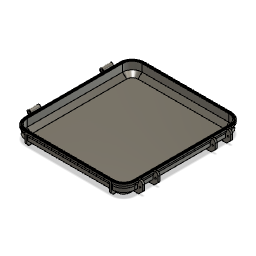
boxw-lid-vii-v14 (Autodesk Fusion 360 design; units mm, degrees)
Autodesk Fusion 360 part; units mm, degrees
sketch "Sketch1" plane through (0, 0, 0) normal (0, 1, 0) x (1, 0, 0)
  line L0 (75.5, -93) -> (-75.5, -93)
  line L1 (-85.5, -83) -> (-85.5, 83)
  line L2 (-75.5, 93) -> (75.5, 93)
  line L3 (85.5, 83) -> (85.5, -83)
  line L4 (85.5, -93) -> (-85.5, 93) construction
  line L5 (-85.5, -93) -> (85.5, 93) construction
  arc A0 (-75.5, 93) -> (-85.5, 83) centre (-75.5, 83) ccw
  arc A1 (85.5, 83) -> (75.5, 93) centre (75.5, 83) ccw
  arc A2 (75.5, -93) -> (85.5, -83) centre (75.5, -83) ccw
  arc A3 (-85.5, -83) -> (-75.5, -93) centre (-75.5, -83) ccw
  dimension "d6" = 186
  dimension "d7" = 171
  dimension "d8" = 10
  dimension "d9" = 10
  dimension "d10" = 10
  dimension "d11" = 10
  constraint horizontal L0
  constraint perpendicular L0 L1
  constraint parallel L0 L2
  constraint parallel L1 L3
  constraint coincident L4 origin
  constraint coincident L5 origin
  constraint coincident L4.end L2
  constraint coincident L4.end L1
  constraint tangent L2 A0
  constraint tangent L1 A0
  constraint coincident L5.end L2
  constraint coincident L5.end L3
  constraint tangent L2 A1
  constraint tangent L3 A1
  constraint coincident L4.start L3
  constraint coincident L4.start L0
  constraint tangent L3 A2
  constraint tangent L0 A2
  constraint coincident L5.start L0
  constraint coincident L5.start L1
  constraint tangent L0 A3
  constraint tangent L1 A3
  measures "d6" distance of L0 L2
  measures "d7" distance of L1 L3
  measures "d8" radius of A0
  measures "d9" radius of A1
  measures "d10" radius of A2
  measures "d11" radius of A3
sketch "Sketch2" plane through (0, 0, 0) normal (0, 0, 1) x (1, 0, 0)
  line L0 (0, 0) -> (85.5, 0)
  line L1 (85.5, 0) -> (85.5, 2.4)
  line L2 (92.5, 9.4) -> (92.5, 22.4)
  line L3 (92.5, 22.4) -> (93.73, 22.4)
  line L4 (93.73, 22.4) -> (93.73, 20.4)
  line L5 (93.73, 20.4) -> (95.53, 20.4)
  line L6 (95.53, 20.4) -> (95.53, 22.4)
  line L7 (95.53, 22.4) -> (96.76, 22.4)
  line L8 (96.76, 22.4) -> (96.76, 19.4)
  line L9 (95.6865, 0) -> (85.5, 0)
  line L10 (96.76, 19.4) -> (94.9, 19.4)
  line L11 (94.9, 19.4) -> (94.9, 15)
  line L12 (94.9, 15) -> (94.9, 8.4059)
  line L13 (94.9, 15) -> (96.76, 19.4)
  line L14 (92.5, 9.4) -> (85.5, 2.4)
  line L15 (86.4941, 0) -> (94.9, 8.4059)
  line L16 (95.6865, 0) -> (103.76, 8.0735)
  line L17 (96.76, 22.4) -> (98.76, 22.4)
  line L18 (103.76, 17.4) -> (103.76, 8.0735)
  arc A0 (103.76, 17.4) -> (98.76, 22.4) centre (98.76, 17.4) ccw
  circle A1 centre (99.26, 12.4) radius 1.425
  line L19 (0, 0) -> (0, 60)
  line L20 (-93.73, 22.4) -> (-93.73, 20.4)
  line L21 (-94.9, 15) -> (-96.76, 19.4)
  line L22 (-92.5, 9.4) -> (-92.5, 22.4)
  line L23 (-85.5, 0) -> (-85.5, 2.4)
  line L24 (-93.73, 20.4) -> (-95.53, 20.4)
  line L25 (-86.4941, 0) -> (-94.9, 8.4059)
  line L26 (-94.9, 15) -> (-94.9, 8.4059)
  line L27 (-92.5, 9.4) -> (-85.5, 2.4)
  line L28 (-96.76, 22.4) -> (-96.76, 19.4)
  line L29 (-94.9, 19.4) -> (-94.9, 15)
  line L30 (-95.53, 22.4) -> (-96.76, 22.4)
  line L31 (-95.53, 20.4) -> (-95.53, 22.4)
  line L32 (-96.76, 19.4) -> (-94.9, 19.4)
  line L33 (-92.5, 22.4) -> (-93.73, 22.4)
  line L34 (94.9, 19.4) -> (92.5, 19.4)
  line L35 (-94.9, 19.4) -> (-92.5, 19.4)
  line L36 (93.73, 22.4) -> (95.53, 22.4)
  line L37 (94.63, 22.4) -> (94.63, 23.3)
  line L38 (99.26, 12.4) -> (99.26, 2.4)
  line L39 (94.63, 23.3) -> (94.83, 23.3)
  line L40 (94.83, 23.3) -> (94.83, 23.06)
  line L41 (94.63, 23.3) -> (94.43, 23.3)
  line L42 (94.43, 23.3) -> (94.43, 23.06)
  line L43 (93.88, 22.4) -> (93.88, 20.4)
  line L44 (95.38, 20.4) -> (95.38, 22.4)
  line L45 (93.88, 22.4) -> (94.63, 23.3)
  line L46 (94.63, 23.3) -> (95.38, 22.4)
  circle A2 centre (-100.36, 22.4) radius 1.675
  circle A3 centre (-100.36, 22.4) radius 3.4
  line L47 (-96.76, 22.4) -> (-96.96, 22.4)
  line L48 (-102.7642, 19.9958) -> (-94.9, 12.1317)
  line L49 (-102.7642, 19.9958) -> (-89.0433, 19.9958) construction
  line L50 (-85.5, 0) -> (-86.4941, 0)
  line L51 (-95.6865, 0) -> (-85.5, 0)
  line L52 (-95.6865, 0) -> (-103.76, 8.0735)
  line L53 (-103.76, 17.4) -> (-103.76, 8.0735)
  line L54 (-103.76, 17.4) -> (-103.76, 22.4)
  line L55 (-100.36, 22.4) -> (-96.76, 22.4)
  point P0 (103.76, 22.4)
  point P1 (-103.76, 22.4)
  dimension "d12" = 85.5
  dimension "d13" = 2.4
  dimension "d15" = 1.23
  dimension "d16" = 2
  dimension "d17" = 1.8
  dimension "d18" = 2
  dimension "d19" = 1.23
  dimension "d20" = 3
  dimension "d23" = 4.4
  dimension "d26" = 2.4
  dimension "d27" = 7
  dimension "d28" = 7
  dimension "d29" = 22.4
  dimension "d30" = 6.5
  dimension "d61" = 7
  dimension "d62" = 5
  dimension "d63" = 2.85
  dimension "d64" = 10
  dimension "d65" = 4.5
  dimension "d124" = 10
  dimension "d134" = 2.4
  dimension "d135" = 0.15
  dimension "d136" = 0.15
  dimension "d137" = 79.611
  dimension "d138" = 0.24
  dimension "d139" = 0.24
  dimension "d156" = 3.35
  dimension "d157" = 3.6
  dimension "d158" = 6.8
  dimension "d159" = 45
  constraint coincident L0.start L19.start
  constraint horizontal L0
  constraint perpendicular L0 L1
  constraint perpendicular L2 L3
  constraint perpendicular L3 L4
  constraint perpendicular L4 L5
  constraint perpendicular L5 L6
  constraint perpendicular L6 L7
  constraint perpendicular L7 L8
  constraint perpendicular L1 L9
  constraint perpendicular L8 L10
  constraint perpendicular L10 L11
  constraint perpendicular L9 L12
  constraint coincident L9 L15.start
  constraint vertical L2
  constraint perpendicular L8 L17
  constraint perpendicular L7 L18
  constraint coincident P0 L17
  constraint coincident P0 L18
  constraint tangent L17 A0
  constraint tangent L18 A0
  constraint perpendicular L0 L19
  constraint symmetric L0.end L19 L23.start
  constraint symmetric L1.end L19 L23.end
  constraint symmetric L2.end L19 L22.end
  constraint symmetric L3.end L19 L20.start
  constraint symmetric L4.end L19 L20.end
  constraint symmetric L5.end L19 L24.end
  constraint symmetric L6.end L19 L30.start
  constraint symmetric L7.end L19 L28.start
  constraint symmetric L8.end L19 L21.end
  constraint symmetric L10.end L19 L29.start
  constraint symmetric L11.end L19 L21.start
  constraint symmetric L2.start L19 L22.start
  constraint symmetric L15.start L19 L25.start
  constraint symmetric L12.end L19 L25.end
  constraint symmetric P0 L19 P1
  constraint coincident L2 L34.end
  constraint perpendicular L2 L34
  constraint coincident L22 L35.end
  constraint perpendicular L22 L35
  constraint midpoint L36 L37.start
  constraint perpendicular L36 L37
  constraint coincident A1.centre L38.start
  constraint vertical L38
  constraint perpendicular L37 L39
  constraint perpendicular L36 L40
  constraint perpendicular L40 L41
  constraint perpendicular L41 L42
  constraint coincident L36 L43.start
  constraint coincident L5 L43.end
  constraint perpendicular L5 L43
  constraint coincident L5 L44.start
  constraint coincident L36 L44.end
  constraint perpendicular L36 L44
  constraint coincident L45 L42.end
  constraint coincident L46 L40.end
  constraint concentric A2 A3
  constraint coincident A3 L47.end
  constraint horizontal L49
  constraint coincident A3 L48.start
  constraint coincident L26 L48.end
  constraint tangent A3 L48
  constraint symmetric L9.start L19 L51.start
  constraint symmetric L16.end L19 L52.end
  constraint symmetric L18.start L19 L53.start
  constraint coincident P1 L54.end
  constraint horizontal L47
  constraint coincident A2.centre A3.centre
  constraint perpendicular L28 L55
  measures "d12" distance of L0.start L0.end
  measures "d13" distance of L0.end L1.end
  measures "d15" distance of L2.end L3.end
  measures "d16" distance of L3.end L4.end
  measures "d17" distance of L4.end L5.end
  measures "d18" distance of L5.end L6.end
  measures "d19" distance of L6.end L7.end
  measures "d20" distance of L7.end L8.end
  measures "d23" distance of L10.end L11.end
  measures "d26" distance of L14 L15
  measures "d27" vertical distance of L1.end L2.start
  measures "d28" horizontal distance of L1.end L2.start
  measures "d29" distance of L0.end L7
  measures "d30" distance of L15 L16
  measures "d61" distance of L7.end P0
  measures "d62" radius of A0
  measures "d63" diameter of A1
  measures "d64" distance of L17 A1.centre
  measures "d65" distance of L18 A1.centre
  measures "d124" distance of A1.centre L38.end
  measures "d134" distance of L2 L12
  measures "d135" distance of L4 L43
  measures "d136" distance of L6 L44
  measures "d137" angle of L45 L46
  measures "d138" distance of L41.end L42.end
  measures "d139" distance of L39.end L40.end
  measures "d156" diameter of A2
  measures "d157" distance of L28.start A2.centre
  measures "d158" diameter of A3
  measures "d159" angle of L48 L49
extrude "Extrude1" add sketch "Sketch1" along normal blind 2.4 makes body 1
sweep "Sweep1" add profiles "Sketch2" path "Sketch1" along A2 L0 A3 L1 A0 L2 A1 L3 section 1 contours L1 L2 L9 L11 L12 L14 L15 L34 | L2 L3 L4 L5 L6 L7 L8 L10 L34 | L10 L11 L13 | L4 L5 L36 L43 | L36 L37 L45 | L5 L36 L43 L44 | L5 L6 L36 L44 | L36 L37 L46 | L41 L42 L45 | L39 L40 L46 separate body makes body 2
ref_plane "WorkPlane2" through (-73.5, 0, 0) normal (1, 0, 0) x (0, 1, 0)
sketch "Sketch4" plane through (-73.5, 0, 0) normal (1, 0, 0) x (0, 0, -1)
  line L0 (0, 0) -> (-93, 0)
  line L1 (-93, 0) -> (-93, 2.4)
  line L2 (-93, 2.4) -> (-100, 2.4)
  line L3 (-100, 2.4) -> (-100, 9.4)
  line L4 (-100, 9.4) -> (-93, 2.4)
  line L5 (-100, 2.4) -> (-100, 5)
  line L6 (-100, 2.4) -> (-100, 19.4)
  line L7 (-100, 19.4) -> (-104.26, 19.4)
  line L8 (-104.26, 19.4) -> (-104.26, 4.4676)
  line L9 (-99.7924, 0) -> (-93, 0)
  line L10 (-99.7924, 0) -> (-104.26, 4.4676)
  line L11 (0, 0) -> (0, 70)
  line L12 (99.7924, 0) -> (104.26, 4.4676)
  line L13 (99.7924, 0) -> (93, 0)
  line L14 (100, 2.4) -> (100, 5)
  line L15 (100, 2.4) -> (100, 19.4)
  line L16 (100, 9.4) -> (93, 2.4)
  line L17 (100, 2.4) -> (100, 9.4)
  line L18 (100, 19.4) -> (104.26, 19.4)
  line L19 (104.26, 19.4) -> (104.26, 4.4676)
  line L20 (93, 0) -> (93, 2.4)
  line L21 (93, 2.4) -> (100, 2.4)
  dimension "d47" = 93
  dimension "d48" = 2.4
  dimension "d49" = 7
  dimension "d50" = 7
  dimension "d52" = 4.26
  dimension "d53" = 6.5
  dimension "d56" = 19.4
  constraint coincident L0.start L11.start
  constraint horizontal L0
  constraint perpendicular L0 L1
  constraint perpendicular L1 L2
  constraint perpendicular L2 L3
  constraint coincident L3 L5.end
  constraint perpendicular L2 L6
  constraint perpendicular L6 L7
  constraint perpendicular L7 L8
  constraint perpendicular L1 L9
  constraint perpendicular L0 L11
  constraint symmetric L0.end L11 L13.end
  constraint symmetric L1.end L11 L16.end
  constraint symmetric L2.end L11 L14.start
  constraint symmetric L3.end L11 L16.start
  constraint symmetric L5.end L11 L14.end
  constraint symmetric L6.end L11 L15.end
  constraint symmetric L7.end L11 L18.end
  constraint symmetric L8.end L11 L12.end
  constraint symmetric L9.start L11 L12.start
  measures "d47" distance of L0.start L0.end
  measures "d48" distance of L0.end L1.end
  measures "d49" distance of L1.end L2.end
  measures "d50" distance of L2.end L3.end
  measures "d52" distance of L6.end L7.end
  measures "d53" distance of L4 L10
  measures "d56" distance of L7 L9
extrude "Extrude2" add sketch "Sketch4" along normal mid plane 3.2 bodies 2 1
ref_plane "WorkPlane3" through (73.5, 0, 0) normal (1, 0, 0) x (0, 1, 0)
sketch "Sketch5" plane through (73.5, 0, 0) normal (1, 0, 0) x (0, 0, -1)
  line L0 (-100, 2.4) -> (-100, 19.4)
  line L1 (-100, 9.4) -> (-93, 2.4)
  line L2 (-93, 2.4) -> (-100, 2.4)
  line L3 (-93, 0) -> (-93, 2.4)
  line L4 (-99.7924, 0) -> (-93, 0)
  line L5 (-99.7924, 0) -> (-104.26, 4.4676)
  line L6 (-104.26, 19.4) -> (-104.26, 4.4676)
  line L7 (-100, 19.4) -> (-104.26, 19.4)
  line L8 (100, 19.4) -> (104.26, 19.4)
  line L9 (104.26, 19.4) -> (104.26, 4.4676)
  line L10 (100, 2.4) -> (100, 19.4)
  line L11 (100, 9.4) -> (93, 2.4)
  line L12 (93, 2.4) -> (100, 2.4)
  line L13 (99.7924, 0) -> (104.26, 4.4676)
  line L14 (93, 0) -> (93, 2.4)
  line L15 (99.7924, 0) -> (93, 0)
extrude "Extrude3" add sketch "Sketch5" along normal mid plane 3.2 bodies 2
ref_plane "WorkPlane4" through (0, 0, -75) normal (0, 0, 1) x (1, 0, 0)
sketch "Sketch6" plane through (0, 0, -75) normal (0, 0, 1) x (1, 0, 0)
  line L0 (96.76, 22.4) -> (98.76, 22.4)
  line L1 (103.76, 17.4) -> (103.76, 8.0735)
  arc A0 (103.76, 17.4) -> (98.76, 22.4) centre (98.76, 17.4) ccw
  line L2 (95.6865, 0) -> (103.76, 8.0735)
  line L3 (95.6865, 0) -> (85.5, 0)
  line L4 (85.5, 0) -> (85.5, 2.4)
  line L5 (92.5, 9.4) -> (85.5, 2.4)
  line L6 (92.5, 9.4) -> (92.5, 22.4)
  line L7 (94.9, 19.4) -> (92.5, 19.4)
  line L8 (96.76, 19.4) -> (94.9, 19.4)
  line L9 (96.76, 22.4) -> (96.76, 19.4)
  circle A1 centre (99.26, 12.4) radius 1.425
  point P0 (103.76, 22.4)
  point P1 (99.26, 12.4)
extrude "Extrude10" add sketch "Sketch6" against normal blind 3.2 bodies 2
ref_plane "WorkPlane5" through (0, 0, -51.4) normal (0, 0, 1) x (1, 0, 0)
sketch "Sketch7" plane through (0, 0, -51.4) normal (0, 0, 1) x (1, 0, 0)
  line L0 (85.5, 0) -> (85.5, 2.4)
  line L1 (92.5, 9.4) -> (85.5, 2.4)
  line L2 (92.5, 9.4) -> (92.5, 22.4)
  line L3 (94.9, 19.4) -> (92.5, 19.4)
  line L4 (96.76, 19.4) -> (94.9, 19.4)
  line L5 (96.76, 22.4) -> (96.76, 19.4)
  line L6 (96.76, 22.4) -> (98.76, 22.4)
  arc A0 (103.76, 17.4) -> (98.76, 22.4) centre (98.76, 17.4) ccw
  line L7 (103.76, 17.4) -> (103.76, 8.0735)
  line L8 (95.6865, 0) -> (103.76, 8.0735)
  line L9 (95.6865, 0) -> (85.5, 0)
  circle A1 centre (99.26, 12.4) radius 1.425
extrude "Extrude11" add sketch "Sketch7" along normal blind 3.2 bodies 2
ref_plane "WorkPlane6" through (0, 0, 75) normal (0, 0, 1) x (1, 0, 0)
sketch "Sketch8" plane through (0, 0, 75) normal (0, 0, 1) x (1, 0, 0)
  line L0 (85.5, 0) -> (85.5, 2.4)
  line L1 (92.5, 9.4) -> (85.5, 2.4)
  line L2 (92.5, 9.4) -> (92.5, 22.4)
  line L3 (94.9, 19.4) -> (92.5, 19.4)
  line L4 (96.76, 19.4) -> (94.9, 19.4)
  line L5 (96.76, 22.4) -> (96.76, 19.4)
  line L6 (96.76, 22.4) -> (98.76, 22.4)
  arc A0 (103.76, 17.4) -> (98.76, 22.4) centre (98.76, 17.4) ccw
  line L7 (103.76, 17.4) -> (103.76, 8.0735)
  line L8 (95.6865, 0) -> (103.76, 8.0735)
  circle A1 centre (99.26, 12.4) radius 1.425
  line L9 (95.6865, 0) -> (85.5, 0)
extrude "Extrude12" add sketch "Sketch8" along normal blind 3.2 bodies 2
ref_plane "WorkPlane7" through (0, 0, 51.4) normal (0, 0, 1) x (1, 0, 0)
sketch "Sketch9" plane through (0, 0, 51.4) normal (0, 0, 1) x (1, 0, 0)
  line L0 (95.6865, 0) -> (103.76, 8.0735)
  line L1 (95.6865, 0) -> (85.5, 0)
  line L2 (103.76, 17.4) -> (103.76, 8.0735)
  arc A0 (103.76, 17.4) -> (98.76, 22.4) centre (98.76, 17.4) ccw
  line L3 (96.76, 22.4) -> (98.76, 22.4)
  line L4 (96.76, 22.4) -> (96.76, 19.4)
  line L5 (96.76, 19.4) -> (94.9, 19.4)
  line L6 (94.9, 19.4) -> (92.5, 19.4)
  line L7 (92.5, 9.4) -> (92.5, 22.4)
  line L8 (92.5, 9.4) -> (85.5, 2.4)
  line L9 (85.5, 0) -> (85.5, 2.4)
  circle A1 centre (99.26, 12.4) radius 1.425
  point P0 (98.76, 17.4)
extrude "Extrude13" add sketch "Sketch9" against normal blind 3.2 bodies 2
ref_plane "WorkPlane8" through (0, 0, -63.2) normal (0, 0, 1) x (1, 0, 0)
sketch "Sketch12" plane through (0, 0, -63.2) normal (0, 0, 1) x (1, 0, 0)
  line L0 (-102.7642, 19.9958) -> (-94.9, 12.1317)
  circle A0 centre (-100.36, 22.4) radius 3.4
  circle A1 centre (-100.36, 22.4) radius 1.675
  line L1 (-96.76, 22.4) -> (-96.96, 22.4)
  line L2 (-96.76, 22.4) -> (-96.76, 19.4)
  line L3 (-94.9, 15) -> (-96.76, 19.4)
  line L4 (-94.9, 15) -> (-94.9, 8.4059)
  line L5 (-103.76, 17.4) -> (-103.76, 8.0735)
  line L6 (-103.76, 17.4) -> (-103.76, 22.4)
  line L7 (-95.6865, 0) -> (-103.76, 8.0735)
  line L8 (-95.6865, 0) -> (-85.5, 0)
  line L9 (-86.4941, 0) -> (-94.9, 8.4059)
extrude "Extrude19" add sketch "Sketch12" along normal mid plane 17.4 contours L0 A0 L1 L2 L3 L4 | A0 bodies 2
extrude "Extrude21" add sketch "Sketch12" along normal mid plane 3.2 contours L0 A0 L4 L5 L6 L7 L8 L9 bodies 2
ref_plane "WorkPlane9" through (0, 0, 63.2) normal (0, 0, 1) x (1, 0, 0)
sketch "Sketch13" plane through (0, 0, 63.2) normal (0, 0, 1) x (1, 0, 0)
  line L0 (-102.7642, 19.9958) -> (-94.9, 12.1317)
  line L1 (-94.9, 15) -> (-96.76, 19.4)
  line L2 (-94.9, 15) -> (-94.9, 8.4059)
  line L3 (-96.76, 22.4) -> (-96.76, 19.4)
  circle A0 centre (-100.36, 22.4) radius 3.4
  circle A1 centre (-100.36, 22.4) radius 1.675
  line L4 (-96.76, 22.4) -> (-96.96, 22.4)
  line L5 (-103.76, 17.4) -> (-103.76, 8.0735)
  line L6 (-103.76, 17.4) -> (-103.76, 22.4)
  line L7 (-95.6865, 0) -> (-103.76, 8.0735)
  line L8 (-95.6865, 0) -> (-85.5, 0)
  line L9 (-86.4941, 0) -> (-94.9, 8.4059)
extrude "Extrude20" add sketch "Sketch13" along normal mid plane 17.4 contours L0 L1 L2 L3 A0 L4 | A0 bodies 2
extrude "Extrude22" add sketch "Sketch13" along normal mid plane 3.2 contours L0 L2 A0 L5 L6 L7 L8 L9 bodies 2
fillet "Fillet2" radius 1 11 faces at (89.5582, 0, 49.2667) (28.5, 0, -27.6667) (-23.9667, 0, 93.3314) (-85.8314, 0, -21.6) (23.9667, 0, -93.3314) (72.9667, 0, 97.8596) (-72.9667, 0, 97.8596) (-92.6224, 0, -63.7333) (-92.6224, 0, 62.6667) (72.9667, 0, -97.8596) (-74.0333, 0, -97.8596) on bodies 2
copy_body "Body->Comp1" bodies 2 removing the originals makes body 3 in component "Box Lid"
component "Box Lid" placed x (1, 0, 0) y (0, 1, 0) z (0, 0, 1) at (0, 0, 0)
equation "width = 185 mm" comment "Min=60"
equation "lengh = 200 mm" comment "Min=120"
equation "hight = 20 mm" comment "Min=20"
equation "d6 = lengh - 14 mm"
equation "d7 = width - 14 mm"
equation "d8 = rcorner"
equation "d9 = rcorner"
equation "d10 = rcorner"
equation "d11 = rcorner"
equation "d12 = width * 0.5 - 7 mm"
equation "d13 = tbox"
equation "d26 = tbox"
equation "d29 = hight + tbox"
equation "d31 = tbox"
equation "d46 = 19 mm - width * 0.5"
equation "d47 = lengh * 0.5 - 7 mm"
equation "d48 = tbox"
equation "d54 = trib / 2"
equation "d56 = hight - 3 mm + tbox"
equation "d57 = width * 0.5 - 19 mm"
equation "d58 = trib / 2"
equation "d60 = phinge - lengh * 0.5"
equation "d63 = screwhole"
equation "d68 = 30 mm - trib * 2"
equation "d71 = lengh * 0.5 - phinge"
equation "d72 = 2 * trib - 30 mm"
equation "d81 = -trib"
equation "d83 = trib"
equation "d85 = trib"
equation "d87 = -trib"
equation "screwhole = 2.85 mm"
equation "rcorner = 10 mm" comment "Min=1 Max=10"
equation "phinge = 25 mm" comment "Position of hinge and latch from lengh dimension"
equation "tbox = 2.4 mm" comment "Min=2.4  Max=4.2 Box thickness"
equation "trib = 3.2 mm" comment "Min=2.4 Max=3.6 Rib thickness"
equation "d134 = tbox + 0.0 mm"
equation "d156 = screwhole + 0.5 mm"
equation "d162 = phinge - lengh / 2 + ( 15 mm - trib )"
equation "d163 = ( 30 mm - trib * 2 - 0.2 mm - 6 mm ) / 2"
equation "d165 = ( lengh / 2 - phinge ) - ( 15 mm - trib )"
equation "d166 = ( 30 mm - trib * 2 - 0.2 mm - 6 mm ) / 2"
equation "d168 = trib / 2"
equation "d170 = trib / 2"
named bodies: "Box Waterproof"
